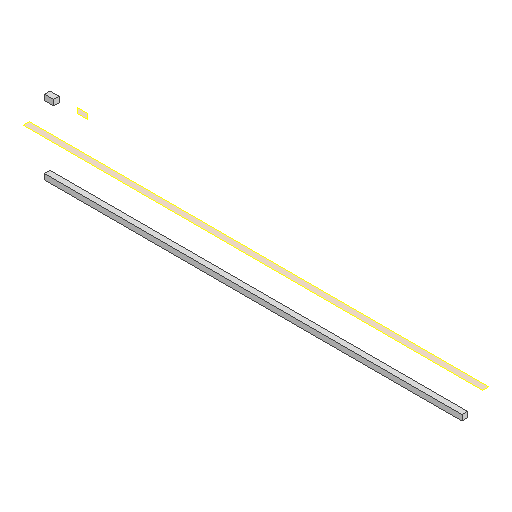
# Autodesk Inventor part: 00_Baseplate_Simmo_side1
Saved by Autodesk Inventor 2022 (Build 260153000, 153)
## iProperties
Created: 2022-04-28
Part Number: 00_Baseplate_Simmo_side1
Material: Generisch
Document SubType Name: Modeling
Designer: diederichbenedict
Density: 1 g/cm^3
Appearance: Vorgabe
Author: diederichbenedict
Autodesk Inventor part; units mm, degrees
ref_plane "YZ Plane" through (0, 0, 0) normal (1, 0, 0) x (0, 1, 0)
ref_plane "XZ Plane" through (0, 0, 0) normal (0, 1, 0) x (-1, 0, 0)
ref_plane "XY Plane" through (0, 0, 0) normal (0, 0, 1) x (1, 0, 0)
ref_plane "Arbeitsebene1" through (0, 0, 0) normal (0, 0, 1) x (1, 0, 0)
sketch "Skizze1" plane through (0, 0, 0) normal (0, 0, 1) x (1, 0, 0)
  line L0 (0, 6) -> (10, 6) projected
  line L1 (10, 0) -> (0, 0) projected
  line L2 (10, 0) -> (10, 6) projected
  line L3 (462.7944, 9) -> (462.7944, 3) projected
  line L4 (0, -68) -> (10, -68) projected
  line L5 (0, 6) -> (450, 6)
  line L6 (450, 6) -> (450, -68)
  line L7 (450, -68) -> (0, -68)
  line L8 (0, -68) -> (0, 6)
  line L9 (0, -68) -> (450, -68)
  line L10 (450, -68) -> (450, -74)
  line L11 (450, -74) -> (0, -74)
  line L12 (0, -74) -> (0, -68)
  line L13 (0, 0) -> (0, 6) projected
  line L14 (129.9001, -74) -> (2.8877, -74) projected
  point P0 (450, 0)
  point P1 (442.7944, 5)
  point P2 (450, -68)
  dimension "d0" = 6
  dimension "d1" = 450
  constraints: 16 end point, 4 parallel, 2 horizontal, 2 perpendicular, 1 point on line
  measures "d0" distance of L9.end L10.end
  measures "d1" distance of L0.start L5.end
extrude "Extrusion1" add sketch "Skizze1" along normal blind 6 contours L0 L2 L1 L8 | L4 L7 L10 L11 L12
sketch "Skizze2" plane through (0, 0, 0) normal (0, 0, -1) x (1, 0, 0)
  line L0 (20, 0) -> (20, -5) projected
  line L1 (10, -5) -> (10, 0) projected
  line L2 (0, -6) -> (0, 74) projected
  line L3 (9.8, -6) -> (20.2, -6)
  line L4 (20.2, -6) -> (20.2, 0)
  line L5 (20.2, 0) -> (9.8, 0)
  line L6 (9.8, 0) -> (9.8, -6)
  point P0 (0, 0)
  dimension "d6" = 0
  dimension "d17" = 0.2
  dimension "d18" = 0.2
  dimension "d23" = 6
  constraints: 8 end point, 2 parallel, 1 horizontal, 1 perpendicular
  measures "d6" distance from line of L1.end L5
  measures "d17" distance between parallel lines of L4 L0
  measures "d18" distance between parallel lines of L6 L1
  measures "d23" distance between parallel lines of L5 L3
extrude "Extrusion2" cut sketch "Skizze2" against normal blind 6
sketch "Skizze3" plane through (20.2, 6, 0) normal (0, 1, 0) x (1, 0, 0)
  line L0 (-10.2, 0) -> (-20.2, 0) projected
  line L1 (-10.2, -6) -> (-20.2, -6) projected
  line L2 (0, 0) -> (0, -6) projected
  circle A0 centre (-5.2, -3) radius 1.5
  line L3 (-10.4, -6) -> (-10.4, 0) projected
  point P0 (4.8, 3)
  point P1 (429.8, 0)
  point P2 (429.8, -6)
  dimension "d16" = 3
  dimension "d19" = 5.2
  constraints: 1 centre point
  measures "d16" diameter of A0
  measures "d19" distance from line of A0.centre L3
hole "Bohrung1" [suppressed]
pattern_linear "Rechteckige Anordnung1" [suppressed]
ref_plane "Arbeitsebene2" through (300.2, -34, 0) normal (0, 1, 0) x (1, 0, 0)
mirror "Spiegeln1" [suppressed]
